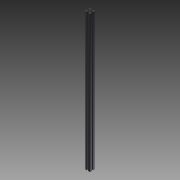
# Autodesk Inventor part: EFS8-4040-1100
Saved by Autodesk Inventor 2015 (Build 190159000, 159)
## iProperties
Category: PARTsolutions
Company: MISUMI
Created: 2015-12-22
Part Number: EFS8-4040-1100
Catalog Web Link: www.cadenas.de
Description: NEFS8-4040, NEFSB8-4040, EFS8-4040, EFSB8-4040, HFS8-4040, HFSB8-4040, CAF8-4040, HFSY8-4040, HFSL8-4040, HFSLB8-4040, GFS8-4040-HFS8 Series Aluminum Extrusions 40 Square -1 Slot-
Vendor: MISUMI
Document SubType Name: Modeling
Designer: psAdmin
Manufacturer: MISUMI
Mass: 659.37 g
Surface Area: 5248.74 cm^2
Volume: 659.37 cm^3
Density: 1 g/cm^3
Material: 一般
Appearance: PSOLRGB-175-175-175
PSOL_IDENT_0: {$CADENAS_DATA\23d-libs\misumi\metric\38_al_extrusions_blackets\8\hfs8_4040.prj},583 {VTYP=3D},{NB=E
PSOL_IDENT_1: FS8-4040-1100},{LINA=EFS8-4040-1100},{NN=NEFS8-4040, NEFSB8-4040, EFS8-4040, EFSB8-4040, HFS8-4040,
PSOL_IDENT_2: HFSB8-4040, CAF8-4040, HFSY8-4040, HFSL8-4040, HFSLB8-4040, GFS8-4040},{DATE=17.07.2015 10:47:41},{G
PSOL_IDENT_3: EOMDATE=28.10.2014 00:00:00},{VERSION=},{LINEID=150},{LINESUBID=-1},{WBVAR=L,ALT1,ALT2,ALT4,ALT5,CP5
PSOL_IDENT_4: ,DL5,DR5,ALT6,ALT9,ALT10,ALT11,HP6,NHL6,DL6,NHR6,DR6,ALT7,ALT8,NH9,AH,BH,CH,DH,EH,NH10,AV,BV,CV,DV,E
PSOL_IDENT_5: V,NH11,AP,BP,CP,DP,EP,ALT12,ALT13,Z,NH12,XA,XB,XC,XD,XE,NH13,YA,YB,YC,YD,YE,ALT14,HP14,DL14,DR14,ALT
PSOL_IDENT_6: 15,HP15,DL15,DR15,ALT16,HP16,DL16,DR16,ALT17,HQ17,JLP,ALT19,ALT20}  {NB=EFS8-4040-1100},{LINA=EFS8-4
PSOL_IDENT_7: 040-1100},{KT=DUMMY},{PN=EFS8-4040-1100},{TPS=EFS8-4040},{MAT=A6N01SS-T5 Aluminum Alloy},{ST=Clear A
PSOL_IDENT_8: nodize},{FRMW=40},{FRMH=40},{FRD=10.5},{L=1100.0},{MASS=1.61},{SA=596},{LX=10.5x10^4},{LY=10.5x10^4}
PSOL_IDENT_9: ,{ALT1=},{M1=0},{IDM1=10.106},{DPL1=0},{DPR1=0},{ALT1PN=},{ALT2=},{ALT2ALG= '','w/o End Tapping (Hel
PSOL_IDENT_10: i-Coil Insert)','LHP','with LHP (Tapping on the Left (Heli-Coil Insert))','RHP','with RHP (Tapping o
PSOL_IDENT_11: n the Right (Heli-Coil Insert))','HPW','with HPW (Tapping on Both Ends (Heli-Coil Insert))' },{M2=0}
PSOL_IDENT_12: ,{DP2=0},{ALT2PN=},{ALT4=},{ALT4ALG= '', 'w/o SC (High Precision Cut)', 'SC', 'with SC (High Precisi
PSOL_IDENT_13: on Cut)' },{ALT4PN=},{ALT5=},{ALT5ALG= '','w/o 45 Degree Cut','1','with 45 Degree Cut' },{CP5=},{CP5
PSOL_IDENT_14: ALG= '','N/A' },{DL5=},{DL5ALG= '','N/A' },{DR5=},{DR5ALG= '','N/A' },{FRMLALT5=0},{FRMRALT5=0},{ALT
PSOL_IDENT_15: 5PN=},{ALT6=},{ALT6ALG= '','w/o Fastening Location Wrench Access Hole Alterations','1','with Fasteni
PSOL_IDENT_16: ng Location Wrench Access Hole Alterations' },{ALT9=},{ALT9ALG= '','w/o Location Specified Wrench Ac
PSOL_IDENT_17: cess Hole Alteratons (Horizontal)','1','with Location Specified Wrench Access Hole Alteratons (Horiz
PSOL_IDENT_18: ontal)' },{ALT10=},{ALT10ALG= '','w/o Location Specified Wrench Access Hole Alteratons (Vertical)','
PSOL_IDENT_19: 1','with Location Specified Wrench Access Hole Alteratons (Vertical)' },{ALT11=},{ALT11ALG= '','w/o
PSOL_IDENT_20: Location Specified Wrench Access Hole Alteratons (Crisscross)','1','with Location Specified Wrench A
PSOL_IDENT_21: ccess Hole Alteratons (Crisscross)' },{HP6=},{HP6ALG= '','N/A' },{NHL6=},{NHL6ALG= '','N/A' },{DL6=}
PSOL_IDENT_22: ,{DL6ALG= '','N/A' },{NHR6=},{NHR6ALG= '','N/A' },{DR6=},{DR6ALG= '','N/A' },{HL6=0},{HL6D=0},{HR6=0
PSOL_IDENT_23: },{HR6D=0},{J6=0},{J6D=0},{K6=0},{K6D=0},{DD6=0},{DD6ALG=0},{ALT7=},{ALT7ALG= '','N/A' },{ALT8=},{AL
PSOL_IDENT_24: T8ALG= '','N/A' },{ALT678PN=},{NH9=0},{NH9MAX=5},{NH9ALG=[0]},{AH=0.0},{AHMIN=7},{AHMAX=1095},{AHALG=
PSOL_IDENT_25: [0]},{BH=0.0},{BHMIN=2},{BHMAX=1097},{BHALG=[0]},{CH=0.0},{CHMIN=2},{CHMAX=1099},{CHALG=[0]},{DH=0.0
PSOL_IDENT_26: },{DHMIN=2},{DHMAX=1101},{DHALG=[0]},{EH=0.0},{EHMIN=2},{EHMAX=1093},{EHALG=[0]},{NH10=0},{NH10MAX=5
PSOL_IDENT_27: },{NH10ALG=[0]},{AV=0.0},{AVMIN=7},{AVMAX=1095},{AVALG=[0]},{BV=0.0},{BVMIN=2},{BVMAX=1097},{BVALG=[
PSOL_IDENT_28: 0]},{CV=0.0},{CVMIN=2},{CVMAX=1099},{CVALG=[0]},{DV=0.0},{DVMIN=2},{DVMAX=1101},{DVALG=[0]},{EV=0.0}
PSOL_IDENT_29: ,{EVMIN=2},{EVMAX=1093},{EVALG=[0]},{NH11=0},{NH11MAX=5},{NH11ALG=[0]},{AP=0.0},{APMIN=7},{APMAX=109
PSOL_IDENT_30: 5},{APALG=[0]},{BP=0.0},{BPMIN=2},{BPMAX=1097},{BPALG=[0]},{CP=0.0},{CPMIN=2},{CPMAX=1099},{CPALG=[0
PSOL_IDENT_31: ]},{DP=0.0},{DPMIN=2},{DPMAX=1101},{DPALG=[0]},{EP=0.0},{EPMIN=2},{EPMAX=1093},{EPALG=[0]},{ALT9PN=}
PSOL_IDENT_32: ,{ALT10PN=},{ALT11PN=},{ALT91011PN=},{ALT12=},{ALT12ALG= '','w/o Counterbore Hole in Specified Posit
PSOL_IDENT_33: ion (Vertical)','1','with Counterbore Hole in Specified Position (Vertical)' },{ALT13=},{ALT13ALG= ''
PSOL_IDENT_34: ,'w/o Counterbore Hole in Specified Position (Horizontal)','1','with Counterbore Hole in Specified P
PSOL_IDENT_35: osition (Horizontal)' },{Z=},{ZALG= '','N/A' },{DD12=0.0},{DD112=0.0},{NH12=0},{NH12MAX=5},{NH12ALG=
PSOL_IDENT_36: [0]},{XA=0.0},{XAMIN=7},{XAMAX=1095},{XAALG=[0]},{XB=0.0},{XBMIN=2},{XBMAX=1097},{XBALG=[0]},{XC=0.0
PSOL_IDENT_37: },{XCMIN=2},{XCMAX=1099},{XCALG=[0]},{XD=0.0},{XDMIN=2},{XDMAX=1101},{XDALG=[0]},{XE=0.0},{XEMIN=2},
PSOL_IDENT_38: {XEMAX=1093},{XEALG=[0]},{NH13=0},{NH13MAX=5},{NH13ALG=[0]},{YA=0.0},{YAMIN=7},{YAMAX=1095},{YAALG=[
PSOL_IDENT_39: 0]},{YB=0.0},{YBMIN=2},{YBMAX=1097},{YBALG=[0]},{YC=0.0},{YCMIN=2},{YCMAX=1099},{YCALG=[0]},{YD=0.0}
PSOL_IDENT_40: ,{YDMIN=2},{YDMAX=1101},{YDALG=[0]},{YE=0.0},{YEMIN=2},{YEMAX=1093},{YEALG=[0]},{ALT12PN=},{ALT13PN=
PSOL_IDENT_41: },{ALT1213PN=},{ALT14=},{ALT14ALG= '','w/o D Type Hole Alteration','1','with D Type Hole Alteration'
PSOL_IDENT_42: },{HP14=},{HP14ALG= '','N/A' },{DL14=},{DL14ALG= '','N/A' },{DR14=},{DR14ALG= '','N/A' },{H14=0},{D
PSOL_IDENT_43: 14=0.0},{ALT14PN=},{ALT15=},{ALT15ALG= '','w/o S Type Hole Alteration','1','with S Type Hole Alterat
PSOL_IDENT_44: ion' },{HP15=},{HP15ALG= '','N/A' },{DL15=},{DL15ALG= '','N/A' },{DR15=},{DR15ALG= '','N/A' },{H15=0
PSOL_IDENT_45: },{D115=0.0},{D215=0.0},{ALT15PN=},{ALT16=},{ALT16ALG= '','w/o M Type Hole Alteration','1','with M T
PSOL_IDENT_46: ype Hole Alteration' },{HP16=},{HP16ALG= '','N/A' },{DL16=},{DL16ALG= '','N/A' },{DR16=},{DR16ALG= ''
PSOL_IDENT_47: ,'N/A' },{H116=0},{D16=0.0},{ALT16PN=},{ALT17=},{ALT17ALG= '','w/o L Type Hole Alteration (Top)','1'
PSOL_IDENT_48: ,'with L Type Hole Alteration (Top)' },{HQ17=0},{HQ17ALG=0},{JLP=0},{JLPMIN=4.9},{JLPMAX=0},{JLPALG=
PSOL_IDENT_49: [0]},{L17=0},{D17=0.0},{ALT17PN=},{ALT19=},{ALT19ALG= '','N/A' },{M19=0},{DP19=0},{ALT19PN=},{ALT20=
PSOL_IDENT_50: },{ALT20PN=},{ERRORALT01=OK},{ERRORALT02=OK},{ERRORALT05=OK},{ERRORALT06091=OK},{ERRORALT06092=OK},{
PSOL_IDENT_51: ERRORALT06093=OK},{ERRORALT06094=OK},{ERRORALT06101=OK},{ERRORALT06102=OK},{ERRORALT06103=OK},{ERROR
PSOL_IDENT_52: ALT06104=OK},{ERRORALT06111=OK},{ERRORALT06112=OK},{ERRORALT06113=OK},{ERRORALT06114=OK},{ERRORALT06
PSOL_IDENT_53: 121=OK},{ERRORALT06122=OK},{ERRORALT06123=OK},{ERRORALT06124=OK},{ERRORALT06131=OK},{ERRORALT06132=O
PSOL_IDENT_54: K},{ERRORALT06133=OK},{ERRORALT06134=OK},{ERRORALT0614=OK},{ERRORALT0615=OK},{ERRORALT0616=OK},{ERRO
PSOL_IDENT_55: RALT06171=OK},{ERRORALT06172=OK},{ERRORALT06173=OK},{ERRORALT0619=OK},{ERRORALT0911=OK},{ERRORALT091
PSOL_IDENT_56: 3=OK},{ERRORALT0914=OK},{ERRORALT0915=OK},{ERRORALT0916=OK},{ERRORALT0917=OK},{ERRORALT0919=OK},{ERR
PSOL_IDENT_57: ORALT1011=OK},{ERRORALT1012=OK},{ERRORALT1014=OK},{ERRORALT1015=OK},{ERRORALT1016=OK},{ERRORALT1017=
PSOL_IDENT_58: OK},{ERRORALT1019=OK},{ERRORALT1112=OK},{ERRORALT1113=OK},{ERRORALT1114=OK},{ERRORALT1115=OK},{ERROR
PSOL_IDENT_59: ALT1116=OK},{ERRORALT1117=OK},{ERRORALT1119=OK},{ERRORALT1214=OK},{ERRORALT1215=OK},{ERRORALT1216=OK
PSOL_IDENT_60: },{ERRORALT1217=OK},{ERRORALT1219=OK},{ERRORALT1314=OK},{ERRORALT1315=OK},{ERRORALT1316=OK},{ERRORAL
PSOL_IDENT_61: T1317=OK},{ERRORALT1319=OK},{ERRORALT1415=OK},{ERRORALT1416=OK},{ERRORALT1417=OK},{ERRORALT1419=OK},
PSOL_IDENT_62: {ERRORALT1516=OK},{ERRORALT1517=OK},{ERRORALT1519=OK},{ERRORALT1617=OK},{ERRORALT1619=OK},{ERRORALT1
PSOL_IDENT_63: 719=OK},{ERRORPN=}
NN: NEFS8-4040, NEFSB8-4040, EFS8-4040, EFSB8-4040, HFS8-4040, HFSB8-4040, CAF8-4040, HFSY8-4040, HFSL8-4040, HFSLB8-4040, GFS8-4040
NT: HFS8 Series Aluminum Extrusions 40 Square -1 Slot-
NB: EFS8-4040-1100
NBSYN: $PN.
LINA: EFS8-4040-1100
PN: EFS8-4040-1100
TPS: EFS8-4040
MAT: A6N01SS-T5 Aluminum Alloy
ST: Clear Anodize
L: 1100.0
MASS: 1.61
SA: 596
LX: 10.5x10^4
LY: 10.5x10^4
ALT1: w/o End Tapping
M1: 0
DPL1: 0
DPR1: 0
ALT2: w/o End Tapping (Heli-Coil Insert)
M2: 0
DP2: 0
ALT4: w/o SC (High Precision Cut)
ALT5: w/o 45 Degree Cut
CP5: N/A
DL5: N/A
DR5: N/A
ALT6: w/o Fastening Location Wrench Access Hole Alterations
ALT9: w/o Location Specified Wrench Access Hole Alteratons (Horizontal)
ALT10: w/o Location Specified Wrench Access Hole Alteratons (Vertical)
ALT11: w/o Location Specified Wrench Access Hole Alteratons (Crisscross)
HP6: N/A
NHL6: N/A
DL6: N/A
NHR6: N/A
DR6: N/A
HL6D: 0
HR6D: 0
J6D: 0
K6D: 0
DD6: 0
ALT7: N/A
ALT8: N/A
NH9: 0
AH: 0.0
BH: 0.0
CH: 0.0
DH: 0.0
EH: 0.0
NH10: 0
AV: 0.0
BV: 0.0
CV: 0.0
DV: 0.0
EV: 0.0
NH11: 0
AP: 0.0
BP: 0.0
CP: 0.0
DP: 0.0
EP: 0.0
ALT12: w/o Counterbore Hole in Specified Position (Vertical)
ALT13: w/o Counterbore Hole in Specified Position (Horizontal)
Z: N/A
DD12: 0.0
DD112: 0.0
NH12: 0
XA: 0.0
XB: 0.0
XC: 0.0
XD: 0.0
XE: 0.0
NH13: 0
YA: 0.0
YB: 0.0
YC: 0.0
YD: 0.0
YE: 0.0
ALT14: w/o D Type Hole Alteration
HP14: N/A
DL14: N/A
DR14: N/A
H14: 0
D14: 0.0
ALT15: w/o S Type Hole Alteration
HP15: N/A
DL15: N/A
DR15: N/A
H15: 0
D115: 0.0
D215: 0.0
ALT16: w/o M Type Hole Alteration
HP16: N/A
DL16: N/A
DR16: N/A
H116: 0
D16: 0.0
ALT17: w/o L Type Hole Alteration (Top)
HQ17: 0
JLP: 0
D17: 0.0
ALT19: N/A
M19: 0
DP19: 0
ALT20: w/o CW (End Face C Chamfering)
SUPPLIER: MISUMI
ARTICLENO: EFS8-4040-1100
BOMINFO: EFS8-4040-1100
CREATOR: CADENAS GmbH
Title: EFS8-4040-1100
Author: Cadenas PARTsolutions
Comments: HFS8 Series Aluminum Extrusions 40 Square -1 Slot-
Autodesk Inventor part; units mm, degrees
sketch "Sketch_2" plane through (0, 0, 0) normal (0, 0, 1) x (1, 0, 0)
  line L0 (-20, 5) -> (-18.2247, 5)
  arc A0 (-18.2247, 5) -> (-17.9882, 5.1154) centre (-18.2247, 5.3) ccw
  arc A1 (-16.4118, 5.1154) -> (-17.9882, 5.1154) centre (-17.2, 4.5) ccw
  arc A2 (-16.4118, 5.1154) -> (-16.1753, 5) centre (-16.1753, 5.3) ccw
  line L1 (-16.1753, 5) -> (-14.5, 5)
  line L2 (-14.5, 5) -> (-14.5, 10)
  line L3 (-14.5, 10) -> (-11.7678, 10)
  line L4 (-11.7678, 10) -> (-7.5, 5.7322)
  line L5 (-7.5, 5.7322) -> (-7.5, 2.4815)
  line L6 (-7.5, 2.4815) -> (-7.2, 1.7)
  line L7 (-7.2, 1.7) -> (-7.4242, 0.6452)
  arc A3 (-7.4242, 0.6452) -> (-7.3681, 0.2912) centre (-6.9351, 0.5412) ccw
  line L8 (-7.3681, 0.2912) -> (-7.2, 0)
  line L9 (-7.2, 0) -> (-7.3681, -0.2912)
  arc A4 (-7.3681, -0.2912) -> (-7.4242, -0.6452) centre (-6.9351, -0.5412) ccw
  line L10 (-7.4242, -0.6452) -> (-7.2, -1.7)
  line L11 (-7.2, -1.7) -> (-7.5, -3.1114)
  line L12 (-7.5, -3.1114) -> (-7.5, -5.7322)
  line L13 (-7.5, -5.7322) -> (-11.7678, -10)
  line L14 (-11.7678, -10) -> (-14.5, -10)
  line L15 (-14.5, -10) -> (-14.5, -5)
  line L16 (-14.5, -5) -> (-16.1753, -5)
  arc A5 (-16.1753, -5) -> (-16.4118, -5.1154) centre (-16.1753, -5.3) ccw
  arc A6 (-17.9882, -5.1154) -> (-16.4118, -5.1154) centre (-17.2, -4.5) ccw
  arc A7 (-17.9882, -5.1154) -> (-18.2247, -5) centre (-18.2247, -5.3) ccw
  line L17 (-18.2247, -5) -> (-20, -5)
  line L18 (-20, -5) -> (-20, -17)
  arc A8 (-20, -17) -> (-17, -20) centre (-17, -17) ccw
  line L19 (-17, -20) -> (-5, -20)
  line L20 (-5, -20) -> (-5, -18.2247)
  arc A9 (-5, -18.2247) -> (-5.1154, -17.9882) centre (-5.3, -18.2247) ccw
  arc A10 (-5.1154, -16.4118) -> (-5.1154, -17.9882) centre (-4.5, -17.2) ccw
  arc A11 (-5.1154, -16.4118) -> (-5, -16.1753) centre (-5.3, -16.1753) ccw
  line L21 (-5, -16.1753) -> (-5, -14.5)
  line L22 (-5, -14.5) -> (-10, -14.5)
  line L23 (-10, -14.5) -> (-10, -11.7678)
  line L24 (-10, -11.7678) -> (-5.7322, -7.5)
  line L25 (-5.7322, -7.5) -> (-2.4815, -7.5)
  line L26 (-2.4815, -7.5) -> (-1.7, -7.2)
  line L27 (-1.7, -7.2) -> (-0.6452, -7.4242)
  arc A12 (-0.6452, -7.4242) -> (-0.2912, -7.3681) centre (-0.5412, -6.9351) ccw
  line L28 (-0.2912, -7.3681) -> (0, -7.2)
  line L29 (0, -7.2) -> (0.2912, -7.3681)
  arc A13 (0.2912, -7.3681) -> (0.6452, -7.4242) centre (0.5412, -6.9351) ccw
  line L30 (0.6452, -7.4242) -> (1.7, -7.2)
  line L31 (1.7, -7.2) -> (3.1114, -7.5)
  line L32 (3.1114, -7.5) -> (5.7322, -7.5)
  line L33 (5.7322, -7.5) -> (10, -11.7678)
  line L34 (10, -11.7678) -> (10, -14.5)
  line L35 (10, -14.5) -> (5, -14.5)
  line L36 (5, -14.5) -> (5, -16.1753)
  arc A14 (5, -16.1753) -> (5.1154, -16.4118) centre (5.3, -16.1753) ccw
  arc A15 (5.1154, -17.9882) -> (5.1154, -16.4118) centre (4.5, -17.2) ccw
  arc A16 (5.1154, -17.9882) -> (5, -18.2247) centre (5.3, -18.2247) ccw
  line L37 (5, -18.2247) -> (5, -20)
  line L38 (5, -20) -> (17, -20)
  arc A17 (17, -20) -> (20, -17) centre (17, -17) ccw
  line L39 (20, -17) -> (20, -5)
  line L40 (20, -5) -> (18.2247, -5)
  arc A18 (18.2247, -5) -> (17.9882, -5.1154) centre (18.2247, -5.3) ccw
  arc A19 (16.4118, -5.1154) -> (17.9882, -5.1154) centre (17.2, -4.5) ccw
  arc A20 (16.4118, -5.1154) -> (16.1753, -5) centre (16.1753, -5.3) ccw
  line L41 (16.1753, -5) -> (14.5, -5)
  line L42 (14.5, -5) -> (14.5, -10)
  line L43 (14.5, -10) -> (11.7678, -10)
  line L44 (11.7678, -10) -> (7.5, -5.7322)
  line L45 (7.5, -5.7322) -> (7.5, -2.4815)
  line L46 (7.5, -2.4815) -> (7.2, -1.7)
  line L47 (7.2, -1.7) -> (7.4242, -0.6452)
  arc A21 (7.4242, -0.6452) -> (7.3681, -0.2912) centre (6.9351, -0.5412) ccw
  line L48 (7.3681, -0.2912) -> (7.2, 0)
  line L49 (7.2, 0) -> (7.3681, 0.2912)
  arc A22 (7.3681, 0.2912) -> (7.4242, 0.6452) centre (6.9351, 0.5412) ccw
  line L50 (7.4242, 0.6452) -> (7.2, 1.7)
  line L51 (7.2, 1.7) -> (7.5, 3.1114)
  line L52 (7.5, 3.1114) -> (7.5, 5.7322)
  line L53 (7.5, 5.7322) -> (11.7678, 10)
  line L54 (11.7678, 10) -> (14.5, 10)
  line L55 (14.5, 10) -> (14.5, 5)
  line L56 (14.5, 5) -> (16.1753, 5)
  arc A23 (16.1753, 5) -> (16.4118, 5.1154) centre (16.1753, 5.3) ccw
  arc A24 (17.9882, 5.1154) -> (16.4118, 5.1154) centre (17.2, 4.5) ccw
  arc A25 (17.9882, 5.1154) -> (18.2247, 5) centre (18.2247, 5.3) ccw
  line L57 (18.2247, 5) -> (20, 5)
  line L58 (20, 5) -> (20, 17)
  arc A26 (20, 17) -> (17, 20) centre (17, 17) ccw
  line L59 (17, 20) -> (5, 20)
  line L60 (5, 20) -> (5, 18.2247)
  arc A27 (5, 18.2247) -> (5.1154, 17.9882) centre (5.3, 18.2247) ccw
  arc A28 (5.1154, 16.4118) -> (5.1154, 17.9882) centre (4.5, 17.2) ccw
  arc A29 (5.1154, 16.4118) -> (5, 16.1753) centre (5.3, 16.1753) ccw
  line L61 (5, 16.1753) -> (5, 14.5)
  line L62 (5, 14.5) -> (10, 14.5)
  line L63 (10, 14.5) -> (10, 11.7678)
  line L64 (10, 11.7678) -> (5.7322, 7.5)
  line L65 (5.7322, 7.5) -> (2.4815, 7.5)
  line L66 (2.4815, 7.5) -> (1.7, 7.2)
  line L67 (1.7, 7.2) -> (0.6452, 7.4242)
  arc A30 (0.6452, 7.4242) -> (0.2912, 7.3681) centre (0.5412, 6.9351) ccw
  line L68 (0.2912, 7.3681) -> (0, 7.2)
  line L69 (0, 7.2) -> (-0.2912, 7.3681)
  arc A31 (-0.2912, 7.3681) -> (-0.6452, 7.4242) centre (-0.5412, 6.9351) ccw
  line L70 (-0.6452, 7.4242) -> (-1.7, 7.2)
  line L71 (-1.7, 7.2) -> (-3.1114, 7.5)
  line L72 (-3.1114, 7.5) -> (-5.7322, 7.5)
  line L73 (-5.7322, 7.5) -> (-10, 11.7678)
  line L74 (-10, 11.7678) -> (-10, 14.5)
  line L75 (-10, 14.5) -> (-5, 14.5)
  line L76 (-5, 14.5) -> (-5, 16.1753)
  arc A32 (-5, 16.1753) -> (-5.1154, 16.4118) centre (-5.3, 16.1753) ccw
  arc A33 (-5.1154, 17.9882) -> (-5.1154, 16.4118) centre (-4.5, 17.2) ccw
  arc A34 (-5.1154, 17.9882) -> (-5, 18.2247) centre (-5.3, 18.2247) ccw
  line L77 (-5, 18.2247) -> (-5, 20)
  line L78 (-5, 20) -> (-17, 20)
  arc A35 (-17, 20) -> (-20, 17) centre (-17, 17) ccw
  line L79 (-20, 17) -> (-20, 5)
  arc A36 (11.05, 17.5) -> (10.5625, 15.6269) centre (11.05, 16.5) ccw
  arc A37 (11.35, 14.5) -> (10.5625, 15.6269) centre (10.15, 14.5) ccw
  line L80 (11.35, 14.5) -> (11.35, 11.85)
  arc A38 (11.35, 11.85) -> (11.85, 11.35) centre (11.85, 11.85) ccw
  line L81 (11.85, 11.35) -> (14.5, 11.35)
  arc A39 (15.6269, 10.5625) -> (14.5, 11.35) centre (14.5, 10.15) ccw
  arc A40 (15.6269, 10.5625) -> (17.5, 11.05) centre (16.5, 11.05) ccw
  line L82 (17.5, 11.05) -> (17.5, 13.9056)
  arc A41 (17.5, 13.9056) -> (17.2071, 14.6127) centre (16.5, 13.9056) ccw
  line L83 (17.2071, 14.6127) -> (14.6127, 17.2071)
  arc A42 (14.6127, 17.2071) -> (13.9056, 17.5) centre (13.9056, 16.5) ccw
  line L84 (13.9056, 17.5) -> (11.05, 17.5)
  arc A43 (10.5625, -15.6269) -> (11.05, -17.5) centre (11.05, -16.5) ccw
  line L85 (11.05, -17.5) -> (13.9056, -17.5)
  arc A44 (13.9056, -17.5) -> (14.6127, -17.2071) centre (13.9056, -16.5) ccw
  line L86 (14.6127, -17.2071) -> (17.2071, -14.6127)
  arc A45 (17.2071, -14.6127) -> (17.5, -13.9056) centre (16.5, -13.9056) ccw
  line L87 (17.5, -13.9056) -> (17.5, -11.05)
  arc A46 (17.5, -11.05) -> (15.6269, -10.5625) centre (16.5, -11.05) ccw
  arc A47 (14.5, -11.35) -> (15.6269, -10.5625) centre (14.5, -10.15) ccw
  line L88 (14.5, -11.35) -> (11.85, -11.35)
  arc A48 (11.85, -11.35) -> (11.35, -11.85) centre (11.85, -11.85) ccw
  line L89 (11.35, -11.85) -> (11.35, -14.5)
  arc A49 (10.5625, -15.6269) -> (11.35, -14.5) centre (10.15, -14.5) ccw
  arc A50 (-17.5, -13.9056) -> (-17.2071, -14.6127) centre (-16.5, -13.9056) ccw
  line L90 (-17.2071, -14.6127) -> (-14.6127, -17.2071)
  arc A51 (-14.6127, -17.2071) -> (-13.9056, -17.5) centre (-13.9056, -16.5) ccw
  line L91 (-13.9056, -17.5) -> (-11.05, -17.5)
  arc A52 (-11.05, -17.5) -> (-10.5625, -15.6269) centre (-11.05, -16.5) ccw
  arc A53 (-11.35, -14.5) -> (-10.5625, -15.6269) centre (-10.15, -14.5) ccw
  line L92 (-11.35, -14.5) -> (-11.35, -11.85)
  arc A54 (-11.35, -11.85) -> (-11.85, -11.35) centre (-11.85, -11.85) ccw
  line L93 (-11.85, -11.35) -> (-14.5, -11.35)
  arc A55 (-15.6269, -10.5625) -> (-14.5, -11.35) centre (-14.5, -10.15) ccw
  arc A56 (-15.6269, -10.5625) -> (-17.5, -11.05) centre (-16.5, -11.05) ccw
  line L94 (-17.5, -11.05) -> (-17.5, -13.9056)
  arc A57 (-17.5, 11.05) -> (-15.6269, 10.5625) centre (-16.5, 11.05) ccw
  arc A58 (-14.5, 11.35) -> (-15.6269, 10.5625) centre (-14.5, 10.15) ccw
  line L95 (-14.5, 11.35) -> (-11.85, 11.35)
  arc A59 (-11.85, 11.35) -> (-11.35, 11.85) centre (-11.85, 11.85) ccw
  line L96 (-11.35, 11.85) -> (-11.35, 14.5)
  arc A60 (-10.5625, 15.6269) -> (-11.35, 14.5) centre (-10.15, 14.5) ccw
  arc A61 (-10.5625, 15.6269) -> (-11.05, 17.5) centre (-11.05, 16.5) ccw
  line L97 (-11.05, 17.5) -> (-13.9056, 17.5)
  arc A62 (-13.9056, 17.5) -> (-14.6127, 17.2071) centre (-13.9056, 16.5) ccw
  line L98 (-14.6127, 17.2071) -> (-17.2071, 14.6127)
  arc A63 (-17.2071, 14.6127) -> (-17.5, 13.9056) centre (-16.5, 13.9056) ccw
  line L99 (-17.5, 13.9056) -> (-17.5, 11.05)
  constraints: 200 end point, 128 point on circle, 64 centre point
extrude "Extrusion1" add sketch "Sketch_2" against normal blind 1100
sketch "Sketch_91" plane through (0, 0, 0) normal (0, 0, 1) x (1, 0, 0)
  line L0 (-6.1, 5.6) -> (-6.1, 2.8)
  arc A0 (-6.1, 2.8) -> (-5.8, 2.5) centre (-5.8, 2.8) ccw
  line L1 (-5.8, 2.5) -> (-5.0953, 2.5)
  arc A1 (-4.8199, 2.0811) -> (-5.0953, 2.5) centre (-5.0953, 2.2) ccw
  arc A2 (-4.8199, 2.0811) -> (-4.8199, -2.0811) centre (0, 0) ccw
  arc A3 (-5.0953, -2.5) -> (-4.8199, -2.0811) centre (-5.0953, -2.2) ccw
  line L2 (-5.0953, -2.5) -> (-5.8, -2.5)
  arc A4 (-5.8, -2.5) -> (-6.1, -2.8) centre (-5.8, -2.8) ccw
  line L3 (-6.1, -2.8) -> (-6.1, -5.6)
  arc A5 (-6.1, -5.6) -> (-5.6, -6.1) centre (-5.6, -5.6) ccw
  line L4 (-5.6, -6.1) -> (-2.8, -6.1)
  arc A6 (-2.8, -6.1) -> (-2.5, -5.8) centre (-2.8, -5.8) ccw
  line L5 (-2.5, -5.8) -> (-2.5, -5.0953)
  arc A7 (-2.0811, -4.8199) -> (-2.5, -5.0953) centre (-2.2, -5.0953) ccw
  arc A8 (-2.0811, -4.8199) -> (2.0811, -4.8199) centre (0, 0) ccw
  arc A9 (2.5, -5.0953) -> (2.0811, -4.8199) centre (2.2, -5.0953) ccw
  line L6 (2.5, -5.0953) -> (2.5, -5.8)
  arc A10 (2.5, -5.8) -> (2.8, -6.1) centre (2.8, -5.8) ccw
  line L7 (2.8, -6.1) -> (5.6, -6.1)
  arc A11 (5.6, -6.1) -> (6.1, -5.6) centre (5.6, -5.6) ccw
  line L8 (6.1, -5.6) -> (6.1, -2.8)
  arc A12 (6.1, -2.8) -> (5.8, -2.5) centre (5.8, -2.8) ccw
  line L9 (5.8, -2.5) -> (5.0953, -2.5)
  arc A13 (4.8199, -2.0811) -> (5.0953, -2.5) centre (5.0953, -2.2) ccw
  arc A14 (4.8199, -2.0811) -> (4.8199, 2.0811) centre (0, 0) ccw
  arc A15 (5.0953, 2.5) -> (4.8199, 2.0811) centre (5.0953, 2.2) ccw
  line L10 (5.0953, 2.5) -> (5.8, 2.5)
  arc A16 (5.8, 2.5) -> (6.1, 2.8) centre (5.8, 2.8) ccw
  line L11 (6.1, 2.8) -> (6.1, 5.6)
  arc A17 (6.1, 5.6) -> (5.6, 6.1) centre (5.6, 5.6) ccw
  line L12 (5.6, 6.1) -> (2.8, 6.1)
  arc A18 (2.8, 6.1) -> (2.5, 5.8) centre (2.8, 5.8) ccw
  line L13 (2.5, 5.8) -> (2.5, 5.0953)
  arc A19 (2.0811, 4.8199) -> (2.5, 5.0953) centre (2.2, 5.0953) ccw
  arc A20 (2.0811, 4.8199) -> (-2.0811, 4.8199) centre (0, 0) ccw
  arc A21 (-2.5, 5.0953) -> (-2.0811, 4.8199) centre (-2.2, 5.0953) ccw
  line L14 (-2.5, 5.0953) -> (-2.5, 5.8)
  arc A22 (-2.5, 5.8) -> (-2.8, 6.1) centre (-2.8, 5.8) ccw
  line L15 (-2.8, 6.1) -> (-5.6, 6.1)
  arc A23 (-5.6, 6.1) -> (-6.1, 5.6) centre (-5.6, 5.6) ccw
  constraints: 48 point on circle, 32 end point, 24 centre point
extrude "Extrusion2" cut sketch "Sketch_91" against normal blind 1100
ref_plane "C1_XY" through (0, 0, 0) normal (0, 0, 1) x (1, 0, 0)
ref_plane "C1_YZ" through (0, 0, 0) normal (1, 0, 0) x (0, 1, 0)
ref_plane "C1_ZX" through (0, 0, 0) normal (0, 1, 0) x (0, 0, 1)
ref_plane "to_frame_cap1_XY" through (0, 0, 0) normal (0, 0, 1) x (1, 0, 0)
ref_plane "to_frame_cap1_YZ" through (0, 0, 0) normal (1, 0, 0) x (0, 1, 0)
ref_plane "to_frame_cap1_ZX" through (0, 0, 0) normal (0, 1, 0) x (0, 0, 1)
ref_plane "to_frame_cap2_XY" through (0, 0, -1100) normal (0, 0, -1) x (1, 0, 0)
ref_plane "to_frame_cap2_YZ" through (0, 0, -1100) normal (1, 0, 0) x (0, -1, 0)
ref_plane "to_frame_cap2_ZX" through (0, 0, -1100) normal (0, -1, 0) x (0, 0, -1)
body "Solid1"
